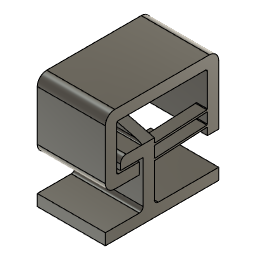
small ver v2 final prototype v2 (Autodesk Fusion 360 design; units mm, degrees)
Autodesk Fusion 360 part; units mm, degrees
sketch "Sketch2" plane through (0, 0, 0) normal (1, 0, 0) x (0, 1, 0)
  line L0 (0, 0) -> (30, 0)
  line L1 (30, 0) -> (30, 30)
  line L2 (30, 30) -> (0, 30)
  line L3 (0, 30) -> (0, 0)
  line L4 (3, 3) -> (27, 3)
  line L5 (27, 3) -> (27, 27)
  line L6 (27, 27) -> (3, 27)
  line L7 (3, 27) -> (3, 3)
  line L8 (13, 3) -> (13, 18.25)
  line L9 (13, 18.25) -> (4, 18.25)
  line L10 (4, 18.25) -> (4, 15.25)
  line L11 (4, 15.25) -> (10, 15.25)
  line L12 (10, 15.25) -> (10, 3)
  line L13 (3, 14.75) -> (9, 14.75)
  line L14 (9, 14.75) -> (9, 11.75)
  line L15 (9, 11.75) -> (3, 11.75)
  line L16 (3, 11.75) -> (0, 11.75)
  line L17 (27, 11.75) -> (30, 11.75)
  line L18 (3, 3) -> (0, 3)
  line L19 (27, 3) -> (30, 3)
  line L20 (13, 13) -> (27, 13.7337)
  line L21 (13, 13.5007) -> (27, 14.2344)
  line L22 (13, 16.5048) -> (27, 17.2385)
  line L23 (13, 17.0055) -> (27, 17.7392)
  point P0 (13, 13)
  dimension "d1" = -3
  dimension "d2" = 30
  dimension "d3" = 30
  dimension "d4" = 3
  dimension "d5" = 3
  dimension "d6" = 3
  dimension "d7" = 0.5
  dimension "d8" = 1
  dimension "d9" = 10
  dimension "d10" = 1
  dimension "d11" = 8.75
  dimension "d91" = 0.5
  dimension "d92" = 0.5
  dimension "d93" = 3
  dimension "d97" = 10
  dimension "d100" = 93
  constraint horizontal L0
  constraint vertical L1
  constraint horizontal L2
  constraint vertical L3
  constraint coincident L0.start L3.end
  constraint coincident L4 L8.start
  constraint perpendicular L4 L8
  constraint perpendicular L8 L9
  constraint perpendicular L9 L10
  constraint perpendicular L10 L11
  constraint coincident L4 L12.end
  constraint perpendicular L4 L12
  constraint perpendicular L7 L13
  constraint perpendicular L4 L14
  constraint coincident L7 L15.end
  constraint perpendicular L7 L15
  constraint coincident L3 L16.end
  constraint perpendicular L3 L16
  constraint coincident L5 L20.end
  constraint coincident L1 L17.end
  constraint perpendicular L1 L17
  constraint coincident L3 L18.end
  constraint perpendicular L3 L18
  constraint coincident L1 L19.end
  constraint perpendicular L1 L19
  constraint coincident L8 P0
  constraint coincident P0 L20.start
  constraint coincident L8 L21.start
  constraint coincident L5 L21.end
  constraint coincident L8 L22.start
  constraint coincident L5 L22.end
  constraint coincident L8 L23.start
  constraint coincident L5 L23.end
  measures "d2" distance of L0.start L2.end
  measures "d3" distance of L1.end L2.end
  measures "d4" distance of L9.end L10.end
  measures "d5" distance of L8 L12
  measures "d6" distance of L13.end L14.end
  measures "d7" distance of L11 L13
  measures "d8" distance of L12 L14
  measures "d9" distance of L3 L12
  measures "d10" distance of L7 L10
  measures "d11" distance of L6 L9
  measures "d91" distance of L22 L23
  measures "d92" distance of L20 L21
  measures "d93" distance of L21 L22
  measures "d97" distance of L4 P0
  measures "d100" angle of L8 L20
extrude "Extrude1" add sketch "Sketch2" along normal blind 18 contours L0 L1 L3 L4 L18 L19 | L1 L2 L3 L5 L6 L7 L16 L17 | L7 L13 L14 L15 | L4 L8 L9 L10 L11 L12 | L5 L8 L20 L21 | L5 L8 L22 L23
sketch "Sketch3" plane through (0, 0, 11.75) normal (0, 0, -1) x (1, 0, 0)
  line L0 (0, 0) -> (0, -9)
  line L1 (0, -9) -> (18, -9)
  line L2 (18, -9) -> (18, 0)
  line L3 (18, 0) -> (0, 0)
  line L4 (9, 0) -> (9, -5.65)
  line L5 (11.65, -8.3) -> (6.35, -8.3)
  line L6 (6.35, -8.3) -> (6.35, -3)
  line L7 (6.35, -3) -> (11.65, -3)
  line L8 (11.65, -3) -> (11.65, -8.3)
  line L9 (11.65, -8.3) -> (6.35, -3) construction
  line L10 (6.35, -8.3) -> (11.65, -3) construction
  point P0 (9, -5.65)
  dimension "d24" = 5.3
  dimension "d25" = 5.3
  dimension "d75" = 3
  constraint midpoint L3 L4.start
  constraint perpendicular L3 L4
  constraint horizontal L5
  constraint perpendicular L5 L6
  constraint parallel L5 L7
  constraint parallel L6 L8
  constraint coincident L9 P0
  constraint coincident L10 P0
  constraint coincident P0 L4.end
  measures "d24" distance of L6.end L7.end
  measures "d25" distance of L5.start L7.end
  measures "d75" distance of L3 L7
extrude "Extrude2" cut sketch "Sketch3" against normal blind 5.3 contours L5 L6 L7 L8
fillet "Fillet1" radius 2.5 3 edges at (9, 0, 30) (9, 30, 30) (9, 0, 11.75)
fillet "Fillet1" radius 0.5 4 edges at (14.825, 3, 14.75) (3.175, 3, 14.75) (9, 27, 27) (9, 3, 27)
fillet "Fillet2" radius 1 2 edges at (9, 10, 3) (9, 13, 3)
sketch "Sketch8" plane through (0, 0, 18.25) normal (0, 0, 1) x (-1, 0, 0)
  line L0 (-18, -4) -> (-18, -13)
  line L1 (-18, -13) -> (0, -13)
  line L2 (0, -13) -> (0, -4)
  line L3 (0, -13) -> (-18, -13)
  line L4 (0, -4) -> (-18, -4)
  line L5 (0, -13) -> (-18, -13)
  line L6 (-18, -13) -> (-18, -10)
  line L7 (-18, -10) -> (0, -10)
  line L8 (0, -10) -> (0, -13)
  dimension "d74" = 3
  constraint horizontal L3
  constraint coincident L1.end L2.start
  constraint horizontal L5
  constraint vertical L6
  constraint horizontal L7
  constraint vertical L8
  constraint coincident L0 L6.end
  measures "d74" distance of L0.end L6.end
extrude "Extrude7" add sketch "Sketch8" along normal blind 2 contours L0 L1 L2 L3 L5 L6 L7 L8
chamfer "Chamfer1" distance 8 distance2 1.99 2 edges at (18, 11.5, 20.25) (0, 11.5, 20.25) measured on face at (12, 11, 20.25) measured on face at (12, 11, 20.25)
fillet "Fillet3" radius 1.5 1 edges at (9, 4, 18.25)
fillet "Fillet4" radius 0.15 6 edges at (9, 13, 13.5007) (9, 27, 14.2344) (9, 27, 17.2385) (9, 27, 17.7392) (9, 13, 17.0055) (9, 13, 16.5048)
fillet "Fillet4" radius 0.15 1 edges at (9, 27, 13.7337)
sketch "Sketch9" plane through (0, 0, 11.75) normal (0, 0, -1) x (1, 0, 0)
  line L0 (0, -27) -> (0, -30)
  line L1 (0, -30) -> (18, -30)
  line L2 (18, -30) -> (18, -27)
  line L3 (18, -27) -> (0, -27)
  line L4 (0, -27) -> (0, -13)
  line L5 (0, -13) -> (18, -13)
  line L6 (18, -13) -> (18, -27)
  line L7 (15, -27) -> (3, -27)
  line L8 (3, -27) -> (3, -13)
  line L9 (3, -13) -> (15, -13)
  line L10 (15, -13) -> (15, -27)
  line L11 (18, -27) -> (0, -27)
  dimension "d64" = 3
  dimension "d65" = 3
  dimension "d96" = 14
  dimension "d101" = 18
  constraint horizontal L3
  constraint vertical L4
  constraint horizontal L5
  constraint vertical L6
  constraint coincident L2.end L3.start
  constraint horizontal L7
  constraint vertical L8
  constraint horizontal L9
  constraint vertical L10
  constraint coincident L5 L8.end
  constraint coincident L3 L7.start
  measures "d64" distance of L6 L10
  measures "d65" distance of L4 L8
  measures "d96" distance of L2.end L5.end
  measures "d101" distance of L4 L6
extrude "Extrude8" cut sketch "Sketch9" along normal blind -10 and the other way blind -1.843 contours L3 L5 L7 L8 L9 L10 L11
extrude "Extrude9" cut 1 faces at (6.35, 6.8667, 16.35) along direction (-1, 0, 0) blind 3
extrude "Extrude10" cut 1 faces at (11.65, 6.8667, 16.35) along direction (1, 0, 0) blind 1.5
extrude "Extrude11" cut 1 faces at (9.8833, 8.3, 16.45) along direction (0, 1, 0) blind 1.5
fillet "Fillet5" radius 0.5 1 edges at (9, 10, 18.25)
sketch "Sketch4" plane through (0, 0, 3) normal (0, 0, 1) x (-1, 0, 0)
  line L0 (0, -9) -> (0, 0)
  line L1 (0, 0) -> (-18, 0)
  line L2 (-18, 0) -> (-18, -9)
  line L3 (-3.5, -10) -> (-14.5, -10)
  line L4 (-14.5, -10) -> (-14.5, 10)
  line L5 (-14.5, 10) -> (-3.5, 10)
  line L6 (-3.5, 10) -> (-3.5, -10)
  line L7 (-3.5, -10) -> (-14.5, 10) construction
  line L8 (-14.5, -10) -> (-3.5, 10) construction
  line L9 (-14.5, -10) -> (-18, -10)
  line L10 (-18, -9) -> (0, -9)
  point P0 (-9, 0)
  dimension "d27" = 11
  dimension "d28" = 20
  constraint horizontal L3
  constraint perpendicular L3 L4
  constraint parallel L3 L5
  constraint parallel L4 L6
  constraint coincident L7 P0
  constraint coincident L8 P0
  constraint midpoint L1 P0
  constraint coincident L2 L9.end
  constraint perpendicular L2 L9
  measures "d27" distance of L3.start L3.end
  measures "d28" distance of L3.end L4.end
extrude "Extrude3" [rolled back] along distance 2.9608 taper angle 0 against distance 4.122 side2taper angle 0
sketch "Sketch5" plane through (0, 0, 3) normal (0, 0, 1) x (-1, 0, 0)
  line L0 (0, -30) -> (0, -14)
  line L1 (-18, -14) -> (-18, -30)
  line L2 (-18, -30) -> (0, -30)
  line L3 (-18, -14) -> (-4, -14)
  line L4 (-4, -14) -> (-4, -30)
  line L5 (-4, -30) -> (-18, -30)
  line L6 (-18, -30) -> (-18, -14)
  line L7 (0, -14) -> (-18, -14)
  dimension "d31" = 14
  constraint horizontal L3
  constraint vertical L4
  constraint horizontal L5
  constraint vertical L6
  constraint coincident L2 L4.end
  constraint coincident L1.start L3.start
  measures "d31" distance of L4.end L1.end
extrude "Extrude4" [rolled back] along distance -5 taper angle 0
